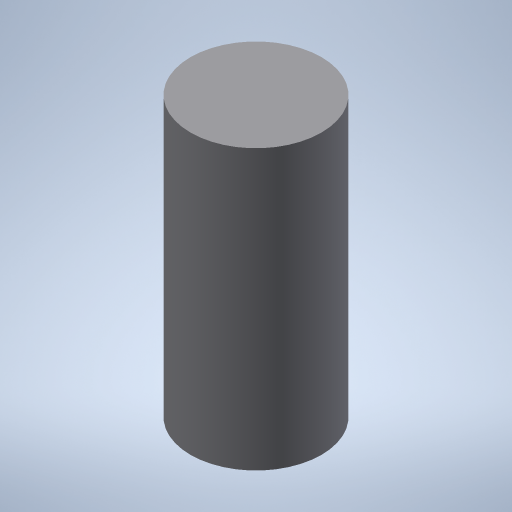
# Autodesk Inventor part: Nema 17 adapter
Saved by Autodesk Inventor 2024 (Build 280153000, 153)
## iProperties
Created: 2012-11-28
Part Number: Nema 17 adapter
Material: Generic
Document SubType Name: Modeling
Designer: Nico
Density: 1 g/cm^3
Appearance: Default
Author: Nico
Autodesk Inventor part; units mm, degrees
ref_plane "YZ Plane" through (0, 0, 0) normal (1, 0, 0) x (0, 1, 0)
ref_plane "XZ Plane" through (0, 0, 0) normal (0, 1, 0) x (-1, 0, 0)
ref_plane "XY Plane" through (0, 0, 0) normal (0, 0, 1) x (1, 0, 0)
sketch "Sketch1" plane through (0, 0, 0) normal (0, 0, 1) x (1, 0, 0)
  line L0 (0, 37.2) -> (5, 42.2)
  line L1 (37.2, 42.2) -> (42.2, 37.2)
  line L2 (42.2, 5) -> (37.2, 0)
  line L3 (5, 0) -> (0, 5)
  line L4 (0, 37.2) -> (0, 5)
  line L5 (37.2, 42.2) -> (5, 42.2)
  line L6 (42.2, 5) -> (42.2, 37.2)
  line L7 (5, 0) -> (37.2, 0)
  line L8 (0, 5) -> (0, 0)
  circle A0 centre (21.1, 21.1) radius 2.5
  circle A1 centre (5.6, 36.6) radius 1.5
  circle A2 centre (36.6, 36.6) radius 1.5
  circle A3 centre (36.6, 5.6) radius 1.5
  circle A4 centre (5.6, 5.6) radius 1.5
  dimension "d8" = 5
  dimension "d9" = 5
  dimension "d10" = 5
  dimension "d11" = 21.1
  dimension "d12" = 21.1
  dimension "d13" = 3
  dimension "d14" = 3
  dimension "d15" = 3
  dimension "d16" = 3
  dimension "d17" = 31
  dimension "d18" = 31
  dimension "d19" = 31
  dimension "d20" = 31
  dimension "d21" = 5.6
  dimension "d22" = 5.6
  dimension "d43" = 5.6
  dimension "d44" = 5.6
  dimension "d45" = 5.6
  dimension "d46" = 5.6
  dimension "d47" = 42.2
  constraints: 18 end point, 5 centre point, 4 parallel, 2 perpendicular, 1 horizontal
  measures "d8" distance of L8.end L3.start
  measures "d9" distance of L8.end L3.end
  measures "d10" diameter of A0
  measures "d11" distance from line of L4 A0.centre
  measures "d12" distance from line of L7 A0.centre
  measures "d13" diameter of A1
  measures "d14" diameter of A2
  measures "d15" diameter of A3
  measures "d16" diameter of A4
  measures "d17" distance of A3.centre A2.centre
  measures "d18" distance of A1.centre A2.centre
  measures "d19" distance of A4.centre A1.centre
  measures "d20" distance of A4.centre A3.centre
  measures "d21" distance from line of L5 A2.centre
  measures "d22" distance from line of L6 A2.centre
  measures "d43" distance from line of L5 A1.centre
  measures "d44" distance from line of L4 A1.centre
  measures "d45" distance from line of L4 A4.centre
  measures "d46" distance from line of L7 A3.centre
  measures "d47" distance between parallel lines of L7 L5
extrude "Extrusion1" add sketch "Sketch1" along normal blind 9.8
sketch "Sketch2" plane through (0, 0, 9.8) normal (0, 0, 1) x (1, 0, 0)
  circle A0 centre (21.1, 21.1) radius 2.5 projected
  circle A1 centre (5.6, 5.6) radius 1.5 projected
  circle A2 centre (36.6, 5.6) radius 1.5 projected
  circle A3 centre (36.6, 36.6) radius 1.5 projected
  circle A4 centre (5.6, 36.6) radius 1.5 projected
  line L0 (5, 42.2) -> (0, 37.2) projected
  line L1 (0, 37.2) -> (0, 5) projected
  line L2 (0, 5) -> (5, 0) projected
  line L3 (5, 0) -> (37.2, 0) projected
  line L4 (37.2, 0) -> (42.2, 5) projected
  line L5 (42.2, 5) -> (42.2, 37.2) projected
  line L6 (42.2, 37.2) -> (37.2, 42.2) projected
  line L7 (37.2, 42.2) -> (5, 42.2) projected
  point P0 (0, 0)
fillet "Fillet1" radius 0.25 8 edges at (21.1, 42.2, 9.8) (39.7, 39.7, 9.8) (42.2, 21.1, 9.8) (39.7, 2.5, 9.8) (21.1, 0, 9.8) (2.5, 2.5, 9.8) (0, 21.1, 9.8) (2.5, 39.7, 9.8)
extrude "Extrusion2" add sketch "Sketch2" along normal blind 31
sketch "Sketch3" plane through (0, 0, 40.8) normal (0, 0, 1) x (1, 0, 0)
  circle A0 centre (21.1, 21.1) radius 2.5 projected
  circle A1 centre (5.6, 36.6) radius 1.5 projected
  circle A2 centre (36.6, 36.6) radius 1.5 projected
  circle A3 centre (36.6, 5.6) radius 1.5 projected
  circle A4 centre (5.6, 5.6) radius 1.5 projected
  line L0 (5, 42.2) -> (0, 37.2) projected
  line L1 (0, 37.2) -> (0, 5) projected
  line L2 (0, 5) -> (5, 0) projected
  line L3 (5, 0) -> (37.2, 0) projected
  line L4 (37.2, 0) -> (42.2, 5) projected
  line L5 (42.2, 5) -> (42.2, 37.2) projected
  line L6 (42.2, 37.2) -> (37.2, 42.2) projected
  line L7 (37.2, 42.2) -> (5, 42.2) projected
  point P0 (0, 0)
fillet "Fillet2" radius 0.25 8 edges at (21.1, 42.2, 40.8) (39.7, 39.7, 40.8) (42.2, 21.1, 40.8) (39.7, 2.5, 40.8) (21.1, 0, 40.8) (2.5, 2.5, 40.8) (0, 21.1, 40.8) (2.5, 39.7, 40.8)
extrude "Extrusion3" add sketch "Sketch3" along normal blind 7.75
sketch "Sketch4" plane through (0, 0, 48.55) normal (0, 0, 1) x (1, 0, 0)
  circle A0 centre (21.1, 21.1) radius 2.5 projected
  circle A1 centre (21.1, 21.1) radius 16
  point P0 (0, 0)
  dimension "d31" = 32
  constraints: 1 centre point, 1 coincident
  measures "d31" diameter of A1
extrude "Extrusion4" cut sketch "Sketch4" against normal blind 0.6
sketch "Sketch5" plane through (21.1, 21.1, 47.95) normal (0, 0, 1) x (1, 0, 0)
  circle A0 centre (0, 0) radius 2.5 projected
  circle A1 centre (0, 0) radius 16 projected
  circle A2 centre (0, 0) radius 11
  point P0 (-21.1, -21.1)
  dimension "d35" = 22
  constraints: 1 centre point, 1 coincident
  measures "d35" diameter of A2
extrude "Extrusion5" add sketch "Sketch5" along normal blind 2.2 contours A2
fillet "Fillet3" radius 0.5 1 edges at (10.1, 21.1, 50.15)
sketch "Sketch6" plane through (21.1, 21.1, 50.15) normal (0, 0, 1) x (1, 0, 0)
  circle A0 centre (0, 0) radius 2.5 projected
  point P0 (-21.1, -21.1)
extrude "Extrusion6" add sketch "Sketch6" along normal blind 22.5
fillet "Fillet4" radius 0.5 1 edges at (18.6, 21.1, 72.65)
sketch "Sketch7" plane through (21.1, 21.1, 72.65) normal (0, 0, 1) x (1, 0, 0)
  circle A0 centre (0, 0) radius 2.6386
  point P0 (-21.1, -21.1)
  constraints: 1 centre point
extrude "Extrusion7" add sketch "Sketch7" along normal blind 15
sketch "Sketch8" plane through (21.1, 21.1, 87.65) normal (0, 0, 1) x (1, 0, 0)
  circle A0 centre (0, 0) radius 2 projected
  circle A1 centre (0, 0) radius 4.7625
  point P0 (-21.1, -21.1)
  dimension "d50" = 9.525
  constraints: 1 centre point, 1 coincident
  measures "d50" diameter of A1
extrude "Extrusion8" add sketch "Sketch8" along normal blind 12.7 contours A0 | A1
sketch "Sketch9" plane through (21.1, 21.1, 87.65) normal (0, 0, -1) x (-1, 0, 0)
  circle A0 centre (0, 0) radius 4.7625 projected
  circle A1 centre (0, 0) radius 2.6386 projected
  point P0 (21.1, -21.1)
extrude "Extrusion9" add sketch "Sketch9" along normal blind 12.7
sketch "Sketch10" plane through (0, 0, 0) normal (0, 0, -1) x (-1, 0, 0)
  circle A0 centre (-21.1, 21.1) radius 2.5 projected
  circle A1 centre (-5.6, 5.6) radius 1.5 projected
  circle A2 centre (-36.6, 5.6) radius 1.5 projected
  circle A3 centre (-36.6, 36.6) radius 1.5 projected
  circle A4 centre (-5.6, 36.6) radius 1.5 projected
  line L0 (0, 37.2) -> (-5, 42.2) projected
  line L1 (-5, 42.2) -> (-37.2, 42.2) projected
  line L2 (-37.2, 42.2) -> (-42.2, 37.2) projected
  line L3 (-42.2, 37.2) -> (-42.2, 5) projected
  line L4 (-42.2, 5) -> (-37.2, 0) projected
  line L5 (-37.2, 0) -> (-5, 0) projected
  line L6 (-5, 0) -> (0, 5) projected
  line L7 (0, 5) -> (0, 37.2) projected
  circle A5 centre (-21.1, 21.1) radius 2 projected
  circle A6 centre (-21.1, 21.1) radius 2.5 projected
  circle A7 centre (-21.1, 21.1) radius 2.5 projected
  point P0 (0, 0)
extrude "Extrusion10" cut sketch "Sketch10" against normal blind 72.8 contours A0 | A1 | A2 | A3 | A4 | L7 L6 L5 L4 L3 L2 L1 L0 | A5
sketch "Sketch12" plane through (21.1, 21.1, 72.8) normal (0, 0, -1) x (-1, 0, 0)
  circle A0 centre (0, 0) radius 2.6386 projected
  point P0 (21.1, -21.1)
extrude "Extrusion11" cut sketch "Sketch12" against normal blind 16.7
sketch "Sketch13" plane through (21.1, 21.1, 100.35) normal (0, 0, 1) x (1, 0, 0)
  circle A0 centre (0, 0) radius 4.7625 projected
  point P0 (-21.1, -21.1)
extrude "Extrusion12" cut sketch "Sketch13" against normal blind 5.08
body "Solid1"
